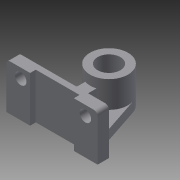
# Autodesk Inventor part: 零件7-19
Saved by Autodesk Inventor 2014 (Build 180170000, 170)
## iProperties
Created: 2018-12-21
Part Number: 零件7-19
Material: 常规
Document SubType Name: Modeling
Designer: Administrator
Density: 1 g/cm^3
Appearance: 默认
Author: Administrator
Autodesk Inventor part; units mm, degrees
ref_plane "YZ Plane" through (0, 0, 0) normal (1, 0, 0) x (0, 1, 0)
ref_plane "XZ Plane" through (0, 0, 0) normal (0, 1, 0) x (-1, 0, 0)
ref_plane "XY Plane" through (0, 0, 0) normal (0, 0, 1) x (1, 0, 0)
sketch "草图1" plane through (0, 0, 0) normal (0, 1, 0) x (-1, 0, 0)
  line L0 (24, 0) -> (-24, 0)
  line L1 (-24, 0) -> (-24, 22)
  line L2 (-22, 24) -> (22, 24)
  line L3 (24, 22) -> (24, 0)
  line L4 (0, 29.295577) -> (0, -8.008859)
  arc A0 (24, 22) -> (22, 24) centre (22, 22) ccw
  arc A1 (-22, 24) -> (-24, 22) centre (-22, 22) ccw
  line L5 (28.197943, 19) -> (-37.870085, 19) construction
  circle A2 centre (16.428853, 19) radius 3
  circle A3 centre (-17.571147, 19) radius 3
  point P0 (0, 0)
  point P1 (-24, 24)
  dimension "d0" = 24
  dimension "d1" = 48
  dimension "d2" = 2
  dimension "d3" = 5
  dimension "d4" = 6
  dimension "d5" = 6
  dimension "d6" = 34
  constraints: 12 end point, 5 point on line, 4 centre point, 4 point on circle, 4 tangent, 3 parallel, 2 perpendicular, 1 equal radius, 1 horizontal, 1 other
  measures "d0" distance of L0.end point (-24, 24)
  measures "d1" distance of L0.start L0.end
  measures "d2" radius of A0
  measures "d3" distance between parallel lines of L2 L5
  measures "d4" diameter of A2
  measures "d5" diameter of A3
  measures "d6" distance of A2.centre A3.centre
extrude "拉伸1" add sketch "草图1" along normal blind 6
sketch "草图2" plane through (0, 0, 0) normal (0, 0, 1) x (1, 0, 0)
  line L0 (22, 0) -> (-22, 0) projected
  line L1 (22, 0) -> (22, 6) projected
  line L2 (-22, 6) -> (22, 6) projected
  line L3 (-22, 0) -> (-22, 6) projected
  line L4 (11.5, -3) -> (-11.5, -3)
  line L5 (-11.5, -3) -> (-11.5, 3)
  line L6 (-11.5, 3) -> (11.5, 3)
  line L7 (11.5, 3) -> (11.5, -3)
  line L8 (11.5, -3) -> (-11.5, 3) construction
  line L9 (-11.5, -3) -> (11.5, 3) construction
  point P0 (0, 0)
  dimension "d9" = 23
  dimension "d10" = 6
  constraints: 12 end point, 2 midpoint, 2 parallel, 1 horizontal, 1 perpendicular
  measures "d9" distance of L5.end L6.end
  measures "d10" distance of L4.end L5.end
extrude "拉伸2" cut sketch "草图2" along normal blind 30 contours L7 L4 L5 L0 | L0 L5 L6 L7
sketch "草图3" plane through (0, 0, 0) normal (0, 0, 1) x (1, 0, 0)
  circle A0 centre (0, 30) radius 10
  line L0 (11.5, 3) -> (11.5, 0)
  line L1 (22, 0) -> (11.5, 0)
  line L2 (22, 0) -> (22, 6)
  line L3 (-22, 6) -> (22, 6)
  line L4 (-22, 0) -> (-22, 6)
  line L5 (-11.5, 0) -> (-22, 0)
  line L6 (-11.5, 0) -> (-11.5, 3)
  line L7 (-11.5, 3) -> (11.5, 3)
  line L8 (0, -6.997144) -> (0, 46.686565)
  circle A1 centre (0, 30) radius 6
  point P0 (0, 0)
  dimension "d13" = 20
  dimension "d14" = 30
  dimension "d15" = 12
  constraints: 2 centre point, 2 end point, 2 point on line, 1 coincident, 1 perpendicular
  measures "d13" diameter of A0
  measures "d14" distance of point (0, 0) A0.centre
  measures "d15" diameter of A1
extrude "拉伸3" add sketch "草图3" along normal blind 19 contours A0 L8 A1 | L8 A1 A0
sketch "草图4" plane through (0, 30, 0) normal (0, 0, -1) x (-1, 0, 0)
  circle A0 centre (0, 0) radius 10
  line L0 (-11.5, -30) -> (-11.5, -27)
  line L1 (-11.5, -27) -> (11.5, -27)
  line L2 (11.5, -27) -> (11.5, -30)
  line L3 (24, -30) -> (11.5, -30)
  line L4 (24, -30) -> (24, -24)
  line L5 (-24, -24) -> (24, -24)
  line L6 (-24, -30) -> (-24, -24)
  line L7 (-11.5, -30) -> (-24, -30)
  line L8 (-9.4744, 3.199335) -> (-18.5, -24)
  line L9 (9.4744, 3.199335) -> (18.5, -24)
  line L10 (0, -31.113393) -> (0, 9.909735)
  point P0 (0, -30)
  dimension "d18" = 37
  constraints: 6 end point, 3 point on line, 2 point on circle, 1 perpendicular, 1 other
  measures "d18" distance of L8.end L9.end
sketch "草图4 outline for 拉伸4" plane through (0, 30, 0) normal (0, 0, -1) x (-1, 0, 0)
  line L0 (18.5, -24) -> (9.4744, 3.199335)
  line L1 (-18.5, -24) -> (18.5, -24)
  line L2 (-9.4744, 3.199335) -> (-18.5, -24)
  arc A0 (-9.4744, 3.199335) -> (9.4744, 3.199335) centre (0, 0) ccw
extrude "拉伸4" add sketch "草图4 outline for 拉伸4" against normal blind 5
sketch "草图5" plane through (0, 30, 5) normal (0, 0, 1) x (1, 0, 0)
  arc A0 (-9.507538, 3.099472) -> (9.507538, 3.099472) centre (0, 0) ccw
  line L0 (18.5, -24) -> (-18.5, -24)
  line L1 (3, -8) -> (-3, -8)
  line L2 (-3, -8) -> (-3, -24)
  line L3 (-3, -24) -> (3, -24)
  line L4 (3, -24) -> (3, -8)
  line L5 (3, -8) -> (-3, -24) construction
  line L6 (-3, -8) -> (3, -24) construction
  line L7 (0, -30) -> (0, 0)
  point P0 (0, -16)
  point P1 (0, -16)
  dimension "d21" = 16
  dimension "d22" = 6
  constraints: 14 end point, 3 midpoint, 3 parallel, 2 point on line, 1 horizontal, 1 perpendicular
  measures "d21" distance of L3.end L1.start
  measures "d22" distance between parallel lines of L2 L4
extrude "拉伸5" add sketch "草图5" along normal blind 9
